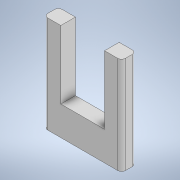
# Autodesk Inventor part: MonofilamentAssemblyJigV1
Saved by Autodesk Inventor 2021 (Build 250183000, 183)
## iProperties
Created: 2021-12-09
Part Number: MonofilamentAssemblyJigV1
Material: Generic
Document SubType Name: Sheet Metal
Designer: Unit-005
Density: 1 g/cm^3
Sheet Metal Rule: Default
Appearance: Default
Author: Unit-005
## iProperties of the stored document _3DPrint.ipt
Created: 2021-12-09
Part Number: _3DPrint
Material: Generic
Document SubType Name: Modeling
Designer: Unit-005
Density: 1 g/cm^3
Appearance: Default
Author: Unit-005
Autodesk Inventor part; units mm, degrees
ref_plane "YZ Plane" through (0, 0, 0) normal (1, 0, 0) x (0, 1, 0)
ref_plane "XZ Plane" through (0, 0, 0) normal (0, 1, 0) x (-1, 0, 0)
ref_plane "XY Plane" through (0, 0, 0) normal (0, 0, 1) x (1, 0, 0)
sketch "Sketch1" plane through (0, 0, 0) normal (0, 0, 1) x (1, 0, 0)
  line L0 (-4, 5) -> (4, 5)
  line L1 (4, 5) -> (4, -5)
  line L2 (4, -5) -> (-4, -5)
  line L3 (-4, -5) -> (-4, 5)
  line L4 (-4, 5) -> (4, -5) construction
  line L5 (4, 5) -> (-4, -5) construction
  point P0 (0, 0)
  dimension "d0" = 8
  dimension "d1" = 10
  constraints: 12 end point, 2 midpoint, 2 parallel, 1 horizontal, 1 perpendicular
  measures "d0" distance of L1.end L2.end
  measures "d1" distance of L0.end L1.end
extrude "Extrusion1" add sketch "Sketch1" along normal blind 1.5
sketch "Sketch2" plane through (0, 0, 1.5) normal (0, 0, 1) x (1, 0, 0)
  line L0 (-4, -5) -> (4, -5) projected
  line L1 (4, -5) -> (4, 5) projected
  line L2 (4, 5) -> (-4, 5) projected
  line L3 (-4, 5) -> (-4, -5) projected
  line L4 (-5.6, 0) -> (5.6, 0) projected
  line L5 (0, -7) -> (0, 7) projected
  line L6 (4, 5) -> (-4, 5) projected
  line L7 (-2.25, 5) -> (2.25, 5)
  line L8 (2.25, 5) -> (2.25, -2)
  line L9 (2.25, -2) -> (-2.25, -2)
  line L10 (-2.25, -2) -> (-2.25, 5)
  point P0 (0, 0)
  dimension "d4" = 4.5
  dimension "d5" = 7
  constraints: 8 end point, 2 parallel, 1 horizontal, 1 perpendicular, 1 point on line, 1 other
  measures "d4" distance of L8.end L9.end
  measures "d5" distance of L7.end L8.end
extrude "Extrusion2" cut sketch "Sketch2" against normal through all contours L9 L10 L4 L5 | L5 L4 L8 L9 | L10 L2 L5 L4 | L5 L2 L8 L4
fillet "Fillet1" radius 0.4 4 edges at (-4, 0, 1.5) (-4, 0, 0) (4, 0, 0) (4, 0, 1.5)
equation "\"BendRadius\" = Thickness"
equation "\"BendReliefWidth\" = Thickness"
equation "\"BendReliefDepth\" = 0.5 * Thickness"
equation "\"CornerReliefSize\" = 4 * Thickness"
equation "\"MinimumRemnant\" = 2 * Thickness"
equation "\"TransitionRadius\" = BendRadius"
equation "\"JacobiRadiusSize\" = BendRadius"
equation "\"GapSize\" = Thickness"
equation "\"Thickness\" = 3.048"
body "Solid1"
